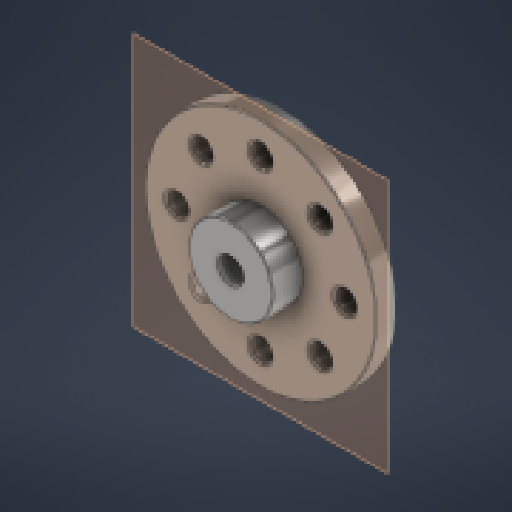
# Autodesk Inventor part: 28Horn
Saved by Autodesk Inventor 2024 (Build 280153000, 153)
## iProperties
Created: 2024-02-15
Part Number: 28Horn
Material: 일반
Document SubType Name: Modeling
Designer: ASUS
Appearance: 강철 - 연마
Surface Area: 10.3617 cm^2
Volume: 0.828027 cm^3
Author: ASUS
Autodesk Inventor part; units mm, degrees
ref_plane "YZ Plane" through (0, 0, 0) normal (1, 0, 0) x (0, 1, 0)
ref_plane "작업 평면1" through (0, 0, 0) normal (0, 0, 1) x (1, 0, 0)
sketch "스케치1" plane through (0, 0, 0) normal (0, 0, 1) x (1, 0, 0)
  circle A0 centre (-8, 0) radius 1 projected
  circle A1 centre (8, 0) radius 1 projected
  circle A2 centre (5.6569, -5.6569) radius 1 projected
  circle A3 centre (-5.6569, 5.6569) radius 1 projected
  circle A4 centre (-5.6569, -5.6569) radius 1 projected
  circle A5 centre (5.6569, 5.6569) radius 1 projected
  circle A6 centre (0, -8) radius 1 projected
  circle A7 centre (0, 8) radius 1 projected
  circle A8 centre (0, 0) radius 4 projected
  circle A9 centre (0, 0) radius 11 projected
  circle A10 centre (0, 0) radius 1.25
  point P0 (0, 0)
  dimension "d0" = 2.5
  constraints: 1 centre point, 1 coincident
  measures "d0" diameter of A10
ref_plane "작업 평면2" through (-11, -11, -2) normal (0, 0, -1) x (0, 1, 0)
extrude "돌출1" add sketch "스케치1" against normal up to surface (2 mm away) contours A8 | A9
sketch "스케치2" plane through (0, 0, 0) normal (0, 0, 1) x (1, 0, 0)
  circle A0 centre (0, 0) radius 2.25 projected
  circle A1 centre (0, 0) radius 4 projected
  circle A2 centre (0, 0) radius 11 projected
  circle A3 centre (-8, 0) radius 1 projected
  circle A4 centre (8, 0) radius 1 projected
  circle A5 centre (5.6569, -5.6569) radius 1 projected
  circle A6 centre (-5.6569, 5.6569) radius 1 projected
  circle A7 centre (-5.6569, -5.6569) radius 1 projected
  circle A8 centre (5.6569, 5.6569) radius 1 projected
  circle A9 centre (0, -8) radius 1 projected
  circle A10 centre (0, 8) radius 1 projected
  circle A11 centre (0, 0) radius 1.25 projected
  point P0 (0, 0)
ref_plane "작업 평면3" through (-4, -4, 2.85) normal (0, 0, 1) x (1, 0, 0)
extrude "돌출2" add sketch "스케치2" along normal up to surface (2.85 mm away) contours A0 | A1
fillet "모깎기1" radius 0.1 3 edges at (-11, 0, 0) (-11, 0, -2) (-4, 0, 2.85)
thread "스레드1" size "M2.5x0.45" class "6H" standard "ANSI Metric M Profile" full length
chamfer "모따기1" distance 0.2 angle 45 8 edges at (-6.6569, 5.6569, 0) (-1, 8, 0) (4.6569, 5.6569, 0) (7, 0, 0) (4.6569, -5.6569, 0) (-1, -8, 0) (-6.6569, -5.6569, 0) (-9, 0, 0)
